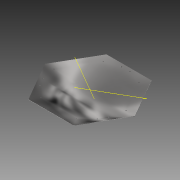
# Autodesk Inventor part: base_bottom
Saved by Autodesk Inventor 2015 SP1 (Build 190203100, 203)
## iProperties
Created: 2015-03-21
Part Number: base_bottom
Material: Ogólny
Document SubType Name: Konstrukcja blachowa
Designer: Marcin
Density: 1 g/cm^3
Appearance: Stal - polerowana
Sheet Metal Rule: Domyślny
Flat Pattern Width: 26 cm
Flat Pattern Length: 30.0222 cm
Flat Pattern Area: 780.578 cm^2
Sheet Metal Width: 260,000 mm
Sheet Metal Length: 300,222 mm
Sheet Metal Area: 78057,756 mm^2
Author: Marcin
Autodesk Inventor part; units mm, degrees
ref_plane "YZ Plane" through (0, 0, 0) normal (1, 0, 0) x (0, 1, 0)
ref_plane "XZ Plane" through (0, 0, 0) normal (0, 1, 0) x (-1, 0, 0)
ref_plane "XY Plane" through (0, 0, 0) normal (0, 0, 1) x (1, 0, 0)
sketch "Szkic1" plane through (0, 0, 0) normal (0, 0, 1) x (1, 0, 0)
  line L0 (75.0555, 130) -> (150.1111, 0)
  line L1 (150.1111, 0) -> (75.0555, -130)
  line L2 (75.0555, -130) -> (-75.0555, -130)
  line L3 (-75.0555, -130) -> (-150.1111, 0)
  line L4 (-150.1111, 0) -> (-75.0555, 130)
  line L5 (-75.0555, 130) -> (75.0555, 130)
  point P0 (0, 0)
  point P1 (0, 0)
  dimension "d0" = 130
  measures "d0" distance from line of L5 point (0, 0)
extrude "Płyta1" add sketch "Szkic1" along normal blind 0.8
ref_plane "Płaszczyzna konstrukcyjna2" through (112.5833, 65, 0.8) normal (-0.5, 0.8660254, 0) x (0, 0, -1)
ref_plane "Płaszczyzna konstrukcyjna3" through (-112.5833, 65, 0) normal (0.5, 0.8660254, 0) x (0, 0, 1)
sketch "Szkic22" plane through (0, 0, 0) normal (0, 0, -1) x (-1, 0, 0)
  circle A0 centre (-120, 0) radius 1.5 projected
  point P0 (0, 0)
  point P1 (-60, -103.923)
  point P2 (60, -103.923)
  point P3 (120, 0)
  point P4 (60, 103.923)
  point P5 (-60, 103.923)
  dimension "d132" = 360
  constraints: 1 coincident, 7 other
hole "Otwór7" at (120, 0, 0) at (60, -103.923, 0) at (-60, -103.923, 0) at (-120, 0, 0) at (-60, 103.923, 0) at (60, 103.923, 0) direction (0, 0, 1) diameter 3 depth 0.8 tip angle 118
sketch "Szkic23" plane through (0, 0, 0) normal (0, 0, -1) x (-1, 0, 0)
  circle A0 centre (-96.057, -71.6244) radius 2 projected
  circle A1 centre (-110.057, -47.3756) radius 2 projected
  line L0 (-106.6109, -41.3446) -> (-89.1109, -71.6554) projected
  line L1 (-89.1109, -71.6554) -> (-99.5032, -77.6554) projected
  line L2 (-117.0032, -47.3446) -> (-99.5032, -77.6554) projected
  line L3 (-106.6109, -41.3446) -> (-117.0032, -47.3446) projected
  circle A2 centre (110.057, -47.3756) radius 2 projected
  circle A3 centre (96.057, -71.6244) radius 2 projected
  line L4 (89.1109, -71.6554) -> (106.6109, -41.3446) projected
  line L5 (106.6109, -41.3446) -> (117.0032, -47.3446) projected
  line L6 (99.5032, -77.6554) -> (117.0032, -47.3446) projected
  line L7 (89.1109, -71.6554) -> (99.5032, -77.6554) projected
  circle A4 centre (-14, 119) radius 2 projected
  circle A5 centre (14, 119) radius 2 projected
  line L8 (17.5, 113) -> (-17.5, 113) projected
  line L9 (-17.5, 113) -> (-17.5, 125) projected
  line L10 (17.5, 125) -> (-17.5, 125) projected
  line L11 (17.5, 113) -> (17.5, 125) projected
  point P0 (0, 0)
  constraints: 6 coincident
hole "Otwór8" at (-96.057, -71.6244, 0) at (-110.057, -47.3756, 0) at (-14, 119, 0) at (14, 119, 0) at (110.057, -47.3756, 0) at (96.057, -71.6244, 0) direction (0, 0, 1) diameter 4 depth 0.8 tip angle 118
equation "\"d139\" = Grubość"
equation "\"d146\" = Grubość"
equation "\"PromieńGięcia\" = Grubość"
equation "\"SzerokośćGięciaPodcięcia\" = Grubość"
equation "\"GłębokośćGięciaPodcięcia\" = 0.5 * Grubość"
equation "\"RozmiarPodcięciaNarożnika\" = 4 * Grubość"
equation "\"MinimalnaPozostałość\" = 2 * Grubość"
equation "\"PromieńPrzejścia\" = PromieńGięcia"
equation "\"Rozmiar_promienia_Jacobiego\" = Grubość"
equation "\"Wielk_odstępu\" = Grubość"
equation "\"d1\" = PromieńGięcia"
equation "\"Grubość\" = 0.8"
